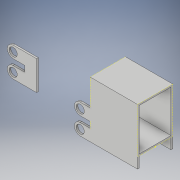
# Autodesk Inventor part: Tape measure holder case Albert
Saved by Autodesk Inventor 2019 (Build 230136000, 136)
## iProperties
Created: 2018-11-07
Part Number: Tape measure holder case Albert
Material: Generic
Document SubType Name: Modeling
Designer: mrhftc
Density: 1 g/cm^3
Appearance: Default
Author: mrhftc
Autodesk Inventor part; units mm, degrees
ref_plane "YZ Plane" through (0, 0, 0) normal (1, 0, 0) x (0, 1, 0)
ref_plane "XZ Plane" through (0, 0, 0) normal (0, 1, 0) x (-1, 0, 0)
ref_plane "XY Plane" through (0, 0, 0) normal (0, 0, 1) x (1, 0, 0)
sketch "Sketch1" plane through (0, 0, 0) normal (0, 1, 0) x (-1, 0, 0)
  line L0 (40.25, 30) -> (-40.25, 30)
  line L1 (-40.25, 30) -> (-40.25, -30)
  line L2 (-40.25, -30) -> (40.25, -30)
  line L3 (40.25, -30) -> (40.25, 30)
  point P0 (0, 0)
  dimension "d0" = 60
  dimension "d1" = 80.5
  dimension "d23" = 30
  dimension "d24" = 40.25
  constraints: 8 end point, 2 parallel, 1 horizontal, 1 perpendicular
  measures "d0" distance of L2.end L0.start
  measures "d1" distance of L0.start L0.end
  measures "d23" distance from line of point (0, 0) L0
  measures "d24" distance from line of point (0, 0) L3
extrude "Extrusion1" add sketch "Sketch1" along normal blind 77.4
sketch "Sketch2" plane through (40.25, 0, 30) normal (1, 0, 0) x (0, 0, -1)
  line L0 (3, 74.4) -> (57, 74.4)
  line L1 (57, 74.4) -> (57, 3)
  line L2 (57, 3) -> (3, 3)
  line L3 (3, 3) -> (3, 74.4)
  line L4 (0, 77.4) -> (60, 77.4) projected
  line L5 (0, 0) -> (0, 77.4) projected
  point P0 (30, 0)
  dimension "d4" = 54
  dimension "d5" = 71.4
  dimension "d6" = 3
  dimension "d7" = 3
  constraints: 8 end point, 2 parallel, 1 horizontal, 1 perpendicular
  measures "d4" distance of L0.start L0.end
  measures "d5" distance of L0.end L1.end
  measures "d6" distance between parallel lines of L4 L0
  measures "d7" distance between parallel lines of L5 L3
sketch "Sketch3" plane through (40.25, 0, 30) normal (1, 0, 0) x (0, 0, -1)
  line L0 (0, 0) -> (60, 0) construction
  line L1 (60, 0) -> (60, 77.4) construction
  line L2 (0, 77.4) -> (60, 77.4) construction
  line L3 (0, 0) -> (0, 77.4) construction
  point P0 (30, 0)
extrude "Extrusion2" cut sketch "Sketch2" against normal blind 74.5
sketch "Sketch4" plane through (-40.25, 0, 30) normal (0, 0, 1) x (1, 0, 0)
  line L0 (0, 12) -> (-17, 12)
  line L1 (-17, 32) -> (0, 32)
  line L2 (0, 32) -> (0, 12)
  line L3 (0, 0) -> (0, 77.4) projected
  line L4 (0, 0) -> (80.5, 0) projected
  circle A0 centre (-17, 22) radius 7
  arc A1 (-17, 32) -> (-17, 12) centre (-17, 22) ccw
  point P0 (40.25, 0)
  dimension "d11" = 20
  dimension "d12" = 0
  dimension "d17" = 14
  dimension "d18" = 22
  dimension "d19" = 20
  dimension "d20" = 17
  constraints: 6 end point, 2 centre point, 2 point on circle, 1 coincident, 1 horizontal, 1 parallel
  measures "d11" distance of L1.end L0.start
  measures "d12" distance between parallel lines of L3 L2
  measures "d17" diameter of A0
  measures "d18" distance from line of L4 A0.centre
  measures "d19" diameter of A1
  measures "d20" distance from line of L2 A0.centre
extrude "Extrusion4" add sketch "Sketch4" against normal blind 3
mirror "Mirror1" about plane through (0, 0, 0) normal (0, 0, 1) of "Extrusion4"
sketch "Sketch7" plane through (-40.25, 0, -30) normal (-1, 0, 0) x (0, 0, 1)
  line L0 (0, 0) -> (60, 0) construction
  line L1 (60, 32) -> (60, 77.4) construction
  line L2 (12.5, 12) -> (47.5, 12)
  line L3 (47.5, 12) -> (47.5, 7)
  line L4 (47.5, 7) -> (12.5, 7)
  line L5 (12.5, 7) -> (12.5, 12)
  point P0 (30, 0)
  dimension "d25" = 35
  dimension "d26" = 5
  dimension "d28" = 12.5
  dimension "d29" = 7
  constraints: 8 end point, 2 parallel, 1 horizontal, 1 perpendicular
  measures "d25" distance of L2.start L2.end
  measures "d26" distance of L2.end L3.end
  measures "d28" distance between parallel lines of L1 L3
  measures "d29" distance between parallel lines of L0 L4
sketch "Sketch8" plane through (-40.25, 0, -30) normal (-1, 0, 0) x (0, 0, 1)
  line L0 (0, 32) -> (3, 32) construction
  line L1 (3, 32) -> (3, 12) construction
  line L2 (3, 12) -> (0, 12) construction
  line L3 (0, 0) -> (0, 12) construction
  line L4 (0, 0) -> (60, 0) construction
  line L5 (60, 0) -> (60, 12) construction
  line L6 (60, 12) -> (57, 12) construction
  line L7 (57, 12) -> (57, 32) construction
  line L8 (57, 32) -> (60, 32) construction
  line L9 (60, 32) -> (60, 77.4) construction
  line L10 (0, 77.4) -> (60, 77.4) construction
  line L11 (0, 32) -> (0, 77.4) construction
  point P0 (30, 0)
extrude "Extrusion6" cut sketch "Sketch7" against normal blind 6
sketch "Sketch10" plane through (40.25, 0, -30) normal (0, 0, -1) x (-1, 0, 0)
  line L0 (80.5, 12) -> (97.5, 12) construction
  line L1 (80.5, 2) -> (97.5, 2)
  line L2 (97.5, 2) -> (97.5, -18)
  line L3 (97.5, -18) -> (80.5, -18)
  line L4 (80.5, -18) -> (80.5, 2)
  circle A0 centre (97.5, -8) radius 10
  arc A1 (97.5, 12) -> (97.5, 32) centre (97.5, 22) ccw construction
  line L5 (80.5, 0) -> (80.5, 12) construction
  point P0 (40.25, 0)
  dimension "d34" = 20
  dimension "d35" = 10
  dimension "d36" = 0
  dimension "d37" = 20
  dimension "d40" = 17
  dimension "d41" = 30
  dimension "d42" = 0
  constraints: 8 end point, 2 parallel, 1 centre point, 1 horizontal, 1 perpendicular
  measures "d34" distance of L1.end L2.end
  measures "d35" distance between parallel lines of L0 L1
  measures "d36" distance from line of L2 A0.centre
  measures "d37" diameter of A0
  measures "d40" distance of L2.end L3.end
  measures "d41" distance of A1.centre A0.centre
  measures "d42" distance between parallel lines of L5 L4
sketch "Sketch13" plane through (40.25, 0, -30) normal (0, 0, -1) x (-1, 0, 0)
  line L0 (0, 0) -> (80.5, 0)
  line L1 (80.5, 0) -> (80.5, -18)
  line L2 (80.5, -18) -> (0, -18)
  line L3 (0, -18) -> (0, 0)
  point P0 (40.25, 0)
  dimension "d43" = 80.5
  dimension "d44" = 18
  constraints: 8 end point, 2 parallel, 1 horizontal, 1 perpendicular
  measures "d43" distance of L1.end L2.end
  measures "d44" distance of L0.end L1.end
extrude "Extrusion8" add sketch "Sketch13" against normal blind 3
extrude "Extrusion9" add sketch "Sketch10" against normal blind 3
sketch "Sketch16" plane through (40.25, 77.4, -30) normal (0, 0, -1) x (-1, 0, 0)
  arc A0 (97.5, -95.4) -> (97.5, -75.4) centre (97.5, -85.4) ccw construction
  circle A1 centre (97.5, -85.4) radius 7
  point P0 (40.25, -77.4)
  dimension "d49" = 14
  constraints: 1 centre point, 1 coincident
  measures "d49" diameter of A1
extrude "Extrusion10" cut sketch "Sketch16" against normal blind 3
mirror "Mirror2" about plane through (0, 0, 0) normal (0, 0, 1) of "Extrusion8", "Extrusion9", "Extrusion10"
sketch "Sketch25" plane through (-40.25, 77.4, 30) normal (0, 0, 1) x (1, 0, 0)
  line L0 (-108.2064, -15.48) -> (-88.2064, -15.48)
  line L1 (-88.2064, -15.48) -> (-88.2064, -65.48)
  line L2 (-88.2064, -65.48) -> (-108.2064, -65.48)
  line L3 (-108.2064, -65.48) -> (-108.2064, -15.48)
  point P0 (40.25, -77.4)
  dimension "d59" = 20
  dimension "d60" = 50
  constraints: 8 end point, 2 parallel, 1 horizontal, 1 perpendicular
  measures "d59" distance of L0.start L0.end
  measures "d60" distance of L0.end L1.end
extrude "Extrusion13" add sketch "Sketch25" along normal blind 3
sketch "Sketch26" plane through (-40.25, 77.4, 33) normal (0, 0, 1) x (1, 0, 0)
  line L0 (-128.2064, -35.48) -> (-108.2064, -35.48)
  line L1 (-108.2064, -35.48) -> (-108.2064, -15.48)
  line L2 (-108.2064, -15.48) -> (-128.2064, -15.48)
  line L3 (-128.2064, -15.48) -> (-128.2064, -35.48)
  line L4 (-108.2064, -65.48) -> (-128.2064, -65.48)
  line L5 (-128.2064, -65.48) -> (-128.2064, -45.48)
  line L6 (-128.2064, -45.48) -> (-108.2064, -45.48)
  line L7 (-108.2064, -45.48) -> (-108.2064, -65.48)
  circle A0 centre (-128.2064, -25.48) radius 10
  circle A1 centre (-128.2064, -55.48) radius 10
  point P0 (40.25, -77.4)
  dimension "d63" = 20
  dimension "d64" = 20
  dimension "d65" = 20
  dimension "d66" = 20
  constraints: 16 end point, 4 parallel, 2 horizontal, 2 midpoint, 2 perpendicular, 2 vertical alignment, 4 other
  measures "d63" distance of L0.start L0.end
  measures "d64" distance of L2.end L0.start
  measures "d65" distance of L5.end L6.end
  measures "d66" distance of L4.end L5.end
extrude "Extrusion14" add sketch "Sketch26" against normal blind 3
sketch "Sketch27" plane through (-40.25, 77.4, 33) normal (0, 0, 1) x (1, 0, 0)
  arc A0 (-128.2064, -15.48) -> (-128.2064, -35.48) centre (-128.2064, -25.48) ccw construction
  arc A1 (-128.2064, -45.48) -> (-128.2064, -65.48) centre (-128.2064, -55.48) ccw construction
  circle A2 centre (-128.2064, -25.48) radius 7
  circle A3 centre (-128.2064, -55.48) radius 7
  point P0 (40.25, -77.4)
  dimension "d69" = 14
  dimension "d70" = 14
  constraints: 2 centre point, 2 coincident
  measures "d69" diameter of A2
  measures "d70" diameter of A3
extrude "Extrusion15" cut sketch "Sketch27" against normal blind 3
body "Solid1"
